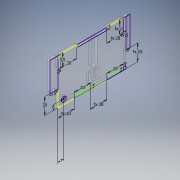
# Autodesk Inventor part: cham_right_v2
Saved by Autodesk Inventor 2017.2 (Build 212233000, 233)
## iProperties
Created: 2017-06-09
Part Number: cham_right_v2
Material: Generic
Document SubType Name: Modeling
Designer: SandeepSH
Density: 1 g/cm^3
Appearance: Polycarbonate - Clear
Author: SandeepSH
Autodesk Inventor part; units mm, degrees
ref_plane "YZ Plane" through (0, 0, 0) normal (1, 0, 0) x (0, 1, 0)
ref_plane "XZ Plane" through (0, 0, 0) normal (0, 1, 0) x (-1, 0, 0)
ref_plane "XY Plane" through (0, 0, 0) normal (0, 0, 1) x (1, 0, 0)
sketch "Sketch1" plane through (0, 0, 0) normal (1, 0, 0) x (0, 1, 0)
  line L0 (0, 0) -> (55.5, 0)
  line L1 (55.5, 0) -> (55.5, -83)
  line L2 (55.5, -83) -> (0, -83)
  line L3 (0, -83) -> (0, 0)
  dimension "d0" = 55.5
  dimension "d1" = 83
  constraints: 8 end point, 2 parallel, 1 horizontal, 1 perpendicular
  measures "d0" distance of L1.end L2.end
  measures "d1" distance of L0.end L1.end
extrude "Extrusion1" add sketch "Sketch1" along normal blind 3
sketch "Sketch2" plane through (3, 0, 0) normal (1, 0, 0) x (0, 0, -1)
  line L0 (20, 0) -> (40, 0)
  line L1 (40, 0) -> (40, 3)
  line L2 (40, 3) -> (20, 3)
  line L3 (20, 3) -> (20, 0)
  line L4 (0, 55.5) -> (0, 0) projected
  line L5 (0, 0) -> (83, 0) projected
  line L6 (60, 0) -> (80, 0)
  line L7 (80, 0) -> (80, 3)
  line L8 (80, 3) -> (60, 3)
  line L9 (60, 3) -> (60, 0)
  line L10 (83, 0) -> (80, 0)
  line L11 (80, 0) -> (80, 3)
  line L12 (80, 3) -> (83, 3)
  line L13 (83, 3) -> (83, 0)
  dimension "d4" = 20
  dimension "d5" = 3
  dimension "d6" = 20
  dimension "d7" = 20
  dimension "d8" = 20
  dimension "d11" = 3
  dimension "d12" = 3
  constraints: 24 end point, 6 parallel, 3 horizontal, 3 perpendicular, 1 point on line
  measures "d4" distance of L2.end L1.end
  measures "d5" distance of L1.end L0.end
  measures "d6" distance between parallel lines of L3 L4
  measures "d7" distance of L8.end L7.end
  measures "d8" distance between parallel lines of L9 L1
  measures "d11" distance of L11.end L12.end
  measures "d12" distance of L10.end L11.end
extrude "Extrusion2" cut sketch "Sketch2" against normal through all contours L3 L2 L1 L0 | L9 L8 L7 L5
extrude "Extrusion3" cut sketch "Sketch2" against normal through all contours L7 L12 L13 L5
sketch "Sketch3" plane through (3, 0, 0) normal (1, 0, 0) x (0, 0, -1)
  point P0 (0, 0)
sketch "Sketch4" plane through (3, 0, 0) normal (1, 0, 0) x (0, 0, -1)
  point P0 (0, 0)
sketch "Sketch5" plane through (3, 0, 0) normal (1, 0, 0) x (0, 0, -1)
  line L0 (0, 0) -> (0, 55.5) projected
  line L1 (0, 55.5) -> (-10, 55.5)
  line L2 (-10, 55.5) -> (-10, 20)
  line L3 (-10, 20) -> (0, 20)
  line L4 (0, 20) -> (0, 55.5)
  line L5 (0, 0) -> (20, 0) projected
  line L6 (83, 55.5) -> (88, 55.5)
  line L7 (88, 55.5) -> (88, 20)
  line L8 (88, 20) -> (83, 20)
  line L9 (83, 20) -> (83, 55.5)
  dimension "d15" = 10
  dimension "d16" = 20
  dimension "d28" = 5
  dimension "d29" = 20
  constraints: 16 end point, 4 parallel, 2 horizontal, 2 perpendicular
  measures "d15" distance of L3.end L2.end
  measures "d16" distance between parallel lines of L5 L3
  measures "d28" distance between parallel lines of L7 L9
  measures "d29" distance between parallel lines of L5 L8
extrude "Extrusion4" add sketch "Sketch5" against normal blind 3 contours L3 L2 L1 L0
sketch "Sketch6" plane through (3, 0, 0) normal (1, 0, 0) x (0, 0, -1)
  line L0 (83, 55.5) -> (-10, 55.5) projected
  line L1 (0, 55.5) -> (3, 55.5)
  line L2 (3, 55.5) -> (3, 40.5)
  line L3 (3, 40.5) -> (0, 40.5)
  line L4 (0, 40.5) -> (0, 55.5)
  line L5 (23, 55.5) -> (60, 55.5)
  line L6 (60, 55.5) -> (60, 52.5)
  line L7 (60, 52.5) -> (23, 52.5)
  line L8 (23, 52.5) -> (23, 55.5)
  line L9 (83, 55.5) -> (80, 55.5)
  line L10 (80, 55.5) -> (80, 40.5)
  line L11 (80, 40.5) -> (83, 40.5)
  line L12 (83, 40.5) -> (83, 55.5)
  point P0 (0, 0)
  dimension "d19" = 3
  dimension "d20" = 15
  dimension "d21" = 3
  dimension "d22" = 20
  dimension "d23" = 3
  dimension "d24" = 15
  dimension "d25" = 20
  constraints: 24 end point, 6 parallel, 3 horizontal, 3 perpendicular, 2 point on line
  measures "d19" distance of L2.end L3.end
  measures "d20" distance of L1.end L2.end
  measures "d21" distance of L5.end L6.end
  measures "d22" distance between parallel lines of L8 L2
  measures "d23" distance between parallel lines of L12 L10
  measures "d24" distance between parallel lines of L11 L0
  measures "d25" distance between parallel lines of L10 L6
extrude "Extrusion5" cut sketch "Sketch6" against normal through all
extrude "Extrusion6" add sketch "Sketch5" against normal blind 3 contours L6 L7 L8 L9
fillet "Fillet1" radius 2 10 edges at (1.5, 55.5, 10) (1.5, 55.5, 0) (1.5, 55.5, -3) (1.5, 20, 10) (1.5, 55.5, -80) (1.5, 55.5, -83) (1.5, 55.5, -88) (1.5, 20, -88) (1.5, 20, -83) (1.5, 20, 0) curvature continuous yes
sketch "Sketch7" plane through (3, 0, 0) normal (1, 0, 0) x (0, 0, -1)
  circle A0 centre (7, 6) radius 3
  line L0 (0, 0) -> (20, 0) projected
  line L1 (0, 18) -> (0, 0) projected
  dimension "d33" = 6
  dimension "d34" = 6
  dimension "d35" = 7
  constraints: 1 centre point
  measures "d33" diameter of A0
  measures "d34" distance from line of L0 A0.centre
  measures "d35" distance from line of L1 A0.centre
extrude "Extrusion7" cut sketch "Sketch7" against normal through all
sketch "Sketch8" plane through (3, 0, 0) normal (1, 0, 0) x (0, 0, -1)
  line L0 (60, 52.5) -> (23, 52.5) projected
  line L1 (41, 52.5) -> (48, 52.5)
  line L2 (48, 52.5) -> (48, 22.5)
  line L3 (48, 22.5) -> (41, 22.5)
  line L4 (41, 22.5) -> (41, 52.5)
  line L5 (0, 18) -> (0, 0) projected
  line L6 (80, 40.5) -> (80, 53.5) projected
  point P0 (44.5, 22.5)
  dimension "d38" = 7
  dimension "d39" = 30
  dimension "d56" = 35.5
  constraints: 8 end point, 2 parallel, 1 horizontal, 1 midpoint, 1 perpendicular, 1 point on line
  measures "d38" distance of L2.end L3.end
  measures "d39" distance of L1.end L2.end
  measures "d56" distance from line of L6 point (44.5, 22.5)
extrude "Extrusion8" cut sketch "Sketch8" against normal through all
sketch "Sketch9" plane through (3, 0, 0) normal (1, 0, 0) x (0, 0, -1)
  line L0 (0, 0) -> (20, 0)
  line L1 (20, 0) -> (20, 3)
  line L2 (20, 3) -> (0, 3)
  line L3 (0, 3) -> (0, 0)
  line L4 (40, 3) -> (40, 0) projected
  line L5 (60, 0) -> (60, 3) projected
  line L6 (40, 0) -> (60, 0)
  line L7 (60, 0) -> (60, 3)
  line L8 (60, 3) -> (40, 3)
  line L9 (40, 3) -> (40, 0)
  constraints: 16 end point, 4 parallel, 2 horizontal, 2 perpendicular
extrude "Extrusion9" cut sketch "Sketch9" against normal through all
sketch "Sketch10" plane through (3, 22, -88) normal (1, 0, 0) x (0, 0, -1)
  line L0 (-45, -4.5) -> (-42, -4.5)
  line L1 (-42, -4.5) -> (-42, -14.5)
  line L2 (-42, -14.5) -> (-45, -14.5)
  line L3 (-45, -14.5) -> (-45, -4.5)
  line L4 (-40, 0.5) -> (-47, 0.5) projected
  line L5 (-43.5, -4.5) -> (-43.5, -0.4579)
  line L6 (-43.5, 0.5) -> (-43.5, 4.5189)
  line L7 (-47, -4.5) -> (-50, -4.5)
  line L8 (-50, -4.5) -> (-50, -14.5)
  line L9 (-50, -14.5) -> (-47, -14.5)
  line L10 (-47, -14.5) -> (-47, -4.5)
  line L11 (-40, -4.5) -> (-37, -4.5)
  line L12 (-37, -4.5) -> (-37, -14.5)
  line L13 (-37, -14.5) -> (-40, -14.5)
  line L14 (-40, -14.5) -> (-40, -4.5)
  point P0 (-88, -22)
  dimension "d45" = 3
  dimension "d46" = 10
  dimension "d47" = 5
  dimension "d48" = 3
  dimension "d49" = 10
  dimension "d50" = 3
  dimension "d51" = 10
  dimension "d52" = 2
  dimension "d53" = 2
  constraints: 28 end point, 6 parallel, 3 horizontal, 3 perpendicular, 2 midpoint, 2 vertical, 1 collinear
  measures "d45" distance of L1.end L2.end
  measures "d46" distance of L0.end L1.end
  measures "d47" distance between parallel lines of L0 L4
  measures "d48" distance of L9.end L8.end
  measures "d49" distance of L8.end L7.end
  measures "d50" distance of L12.end L13.end
  measures "d51" distance of L11.end L12.end
  measures "d52" distance between parallel lines of L3 L10
  measures "d53" distance between parallel lines of L14 L1
extrude "Extrusion10" cut sketch "Sketch10" against normal through all
equation "\"d6\" = d4"
equation "\"d8\" = d6"
equation "\"d29\" = d16"
equation "\"d23\" = d19"
equation "\"d24\" = d20"
equation "\"d25\" = d22"
equation "\"d53\" = d52"
body "Solid1"
